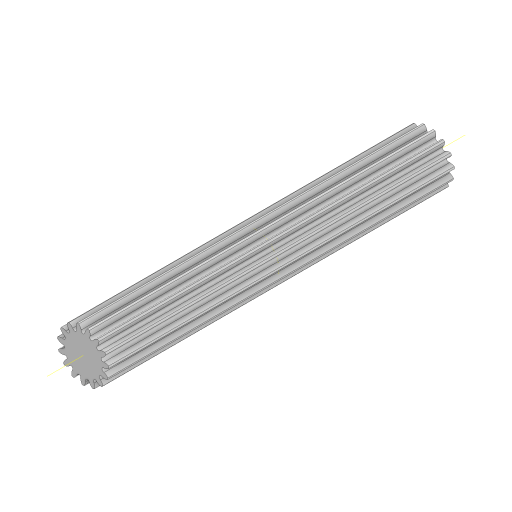
# Autodesk Inventor part: teeth gear 1
Saved by Autodesk Inventor 2024 (Build 280153000, 153)
## iProperties
Created: 2023-05-23
Part Number: teeth gear 1
Material: Generic
Document SubType Name: Modeling
Designer: pc
Density: 1 g/cm^3
Appearance: Default
Author: pc
Autodesk Inventor part; units mm, degrees
ref_plane "YZ Plane" through (0, 0, 0) normal (1, 0, 0) x (0, 1, 0)
ref_plane "XZ Plane" through (0, 0, 0) normal (0, 1, 0) x (-1, 0, 0)
ref_plane "XY Plane" through (0, 0, 0) normal (0, 0, 1) x (1, 0, 0)
sketch "Sketch1" plane through (0, 0, 0) normal (0, 0, 1) x (1, 0, 0)
  spline S0 degree 3 poles (-5.7799, 33.5051) (-5.5975, 33.3106) (-5.2327, 32.9216) (-4.7201, 32.3072) (-4.2357, 31.6704) (-3.7864, 31.0083) (-3.3769, 30.3208) (-3.0754, 29.7257) (-2.8642, 29.236) (-2.7248, 28.8611) (-2.6028, 28.4797) (-2.5539, 28.2174) (-2.5295, 28.0863) knots 0 0 0 0 0.079978 0.159956 0.239933 0.319908 0.39988 0.479846 0.519836 0.559824 0.599809 0.639773 0.639773 0.639773 0.639773
  spline S1 degree 3 poles (-2.5295, 28.0863) (-2.5173, 27.8981) (-2.499, 27.6158) (-2.4421, 27.2428) (-2.3798, 26.9668) (-2.3038, 26.6942) (-2.2029, 26.4297) (-2.0853, 26.1722) (-1.9398, 25.929) (-1.7698, 25.7023) (-1.5732, 25.4981) (-1.3512, 25.3216) (-1.1064, 25.1781) (-0.8426, 25.0734) (-0.5658, 25.0099) (-0.2826, 24.996) (0, 25.002) (0.2826, 24.996) (0.5658, 25.0099) (0.8426, 25.0734) (1.1064, 25.1781) (1.3512, 25.3216) (1.5732, 25.4981) (1.7698, 25.7023) (1.9398, 25.929) (2.0853, 26.1722) (2.2029, 26.4297) (2.3038, 26.6942) (2.3798, 26.9668) (2.4421, 27.2428) (2.499, 27.6158) (2.5173, 27.8981) (2.5295, 28.0863) knots 0 0 0 0 0.056544 0.084824 0.1131 0.141382 0.169655 0.197931 0.226212 0.254488 0.282759 0.31103 0.339307 0.367577 0.395839 0.424093 0.452372 0.480651 0.508905 0.537167 0.565438 0.593714 0.621985 0.650256 0.678532 0.706813 0.735089 0.763363 0.791644 0.819921 0.8482 0.904744 0.904744 0.904744 0.904744
  spline S2 degree 3 poles (2.5295, 28.0863) (2.5539, 28.2174) (2.6028, 28.4797) (2.7248, 28.8611) (2.8642, 29.236) (3.0754, 29.7257) (3.3769, 30.3208) (3.7864, 31.0083) (4.2357, 31.6704) (4.7201, 32.3072) (5.2327, 32.9216) (5.5975, 33.3106) (5.7799, 33.5051) knots 0 0 0 0 0.039964 0.079949 0.119937 0.159926 0.239893 0.319865 0.39984 0.479817 0.559795 0.639773 0.639773 0.639773 0.639773
  circle A0 centre (0, 0) radius 25 construction
  circle A1 centre (0, 0) radius 28.1908 construction
  circle A2 centre (0, 0) radius 30 construction
  circle A3 centre (0, 0) radius 34
  point P0 (-5.2385, 32.9165)
  point P1 (-4.7248, 32.3035)
  point P2 (-4.2416, 31.6662)
  point P3 (-3.793, 31.0041)
  point P4 (-3.3848, 30.3164)
  point P5 (-3.0251, 29.6022)
  point P6 (-2.8674, 29.2347)
  point P7 (-2.7277, 28.86)
  point P8 (-2.6109, 28.4776)
  point P9 (-2.4821, 27.5229)
  point P10 (-2.4388, 27.2434)
  point P11 (-2.3775, 26.9674)
  point P12 (-2.2996, 26.6955)
  point P13 (-2.2001, 26.4309)
  point P14 (-2.0806, 26.1746)
  point P15 (-1.9357, 25.9317)
  point P16 (-1.7654, 25.706)
  point P17 (-1.569, 25.5027)
  point P18 (-1.3474, 25.3271)
  point P19 (-1.1032, 25.1845)
  point P20 (-0.8404, 25.0803)
  point P21 (-0.5647, 25.0182)
  point P22 (-0.2828, 24.9993)
  point P23 (0, 25)
  point P24 (0.2828, 24.9993)
  point P25 (0.5647, 25.0182)
  point P26 (0.8404, 25.0803)
  point P27 (1.1032, 25.1845)
  point P28 (1.3474, 25.3271)
  point P29 (1.569, 25.5027)
  point P30 (1.7654, 25.706)
  point P31 (1.9357, 25.9317)
  point P32 (2.0806, 26.1746)
  point P33 (2.2001, 26.4309)
  point P34 (2.2996, 26.6955)
  point P35 (2.3775, 26.9674)
  point P36 (2.4388, 27.2434)
  point P37 (2.4821, 27.5229)
  point P38 (2.6109, 28.4776)
  point P39 (2.7277, 28.86)
  point P40 (2.8674, 29.2347)
  point P41 (3.0251, 29.6022)
  point P42 (3.3848, 30.3164)
  point P43 (3.793, 31.0041)
  point P44 (4.2416, 31.6662)
  point P45 (4.7248, 32.3035)
  point P46 (5.2385, 32.9165)
  constraints: 4 centre point, 2 point on circle, 109 other
extrude "Extrusion1" add sketch "Sketch1" against normal blind 457.2
extrude "Extrusion2" cut sketch "Sketch1" against normal through all fills toward (-3.751, 31.0311) open curves S0 S1 S2
pattern_circular "Circular Pattern1" count 15 over 360 about axis through (0, 0, 0) along (0, 0, -1) of "Extrusion2"
ref_plane "Work Plane1" through (14.4623, -24.2091, -228.6) normal (0, 0, 1) x (1, 0, 0)
sketch "Sketch3" plane through (14.4623, -24.2091, -228.6) normal (0, 0, 1) x (1, 0, 0)
  circle A0 centre (-14.4623, 24.2091) radius 30 construction
equation "\"d0\" = FaceWidth"
equation "\"Module\" = 4"
equation "\"PressureAngle\" = 20deg"
equation "\"UnitProfileClearance\" = 0.25"
equation "\"UnitRoundRadius\" = 0.35"
equation "\"HeadDiameter\" = 68"
equation "\"RootDiameter\" = 50"
equation "\"BaseDiameter\" = 56.38156"
equation "\"PitchDiameter\" = 60"
equation "\"FaceWidth\" = 457.2"
equation "\"HelixAngle\" = 0"
equation "\"UnitCorrection\" = 0"
equation "\"UnitAddendumModification\" = 0"
equation "\"CircularPitch\" = 12.56637"
equation "\"UnitBacklashShift\" = 0"
equation "\"TotalToolShift\" = 0"
equation "\"IsInternal\" = 0"
body "Solid1"
